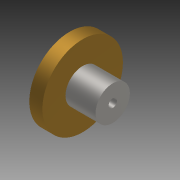
# Autodesk Inventor part: Hitec HS-225MG gear 4
Saved by Autodesk Inventor 2017 SP1 (Build 210196100, 196)
## iProperties
Created: 2018-01-04
Part Number: Hitec HS-225MG gear 4
Material: Generic
Document SubType Name: Modeling
Designer: JT
Density: 1 g/cm^3
Appearance: Default
Author: JT
Autodesk Inventor part; units mm, degrees
ref_plane "YZ Plane" through (0, 0, 0) normal (1, 0, 0) x (0, 1, 0)
ref_plane "XZ Plane" through (0, 0, 0) normal (0, 1, 0) x (-1, 0, 0)
ref_plane "XY Plane" through (0, 0, 0) normal (0, 0, 1) x (1, 0, 0)
sketch "Sketch1" plane through (0, 0, 0) normal (0, 0, 1) x (1, 0, 0)
  line L0 (0.34, 5.75) -> (2.2, 5.75)
  line L1 (2.2, 5.75) -> (2.2, 2.45)
  line L2 (2.2, 2.45) -> (6.5, 2.45)
  line L3 (6.5, 2.45) -> (6.5, 0)
  line L4 (6.5, 0) -> (0, 0)
  line L5 (0, 0) -> (0, 2)
  line L6 (0, 2) -> (0.34, 2)
  line L7 (0.34, 2) -> (0.34, 5.75)
  dimension "d2" = 4.9
  dimension "d3" = 11.5
  dimension "d4" = 1.86
  dimension "d5" = 4
  dimension "d6" = 4.3
  dimension "d7" = 6.5
  constraints: 16 end point, 6 perpendicular, 1 horizontal, 1 vertical
  measures "d2" diameter of L2 L4
  measures "d3" diameter of L0 L4
  measures "d4" distance between parallel lines of L1 L7
  measures "d5" diameter of L6 L4
  measures "d6" distance between parallel lines of L3 L1
  measures "d7" distance between parallel lines of L3 L5
revolve "Revolution1" add sketch "Sketch1" angle 360 about axis through (6.5, 0, 0) along (-1, 0, 0)
hole "Hole1" at (6.5, 0, 0) direction (-1, 0, 0) diameter 1.2 end through all
body "Solid1"
